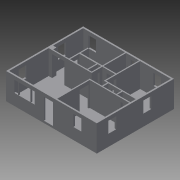
# Autodesk Inventor part: First Floor
Saved by Autodesk Inventor 2013 (Build 170138000, 138)
## iProperties
Created: 2013-06-17
Part Number: First Floor
Material: Generic
Document SubType Name: Modeling
Designer: Joey
Density: 1 g/cm^3
Author: Joey
Autodesk Inventor part; units mm, degrees
ref_plane "YZ Plane" through (0, 0, 0) normal (1, 0, 0) x (0, 1, 0)
ref_plane "XZ Plane" through (0, 0, 0) normal (0, 1, 0) x (-1, 0, 0)
ref_plane "XY Plane" through (0, 0, 0) normal (0, 0, 1) x (1, 0, 0)
sketch "Sketch1" plane through (0, 0, 0) normal (0, 1, 0) x (-1, 0, 0)
  line L0 (6400.8, 0) -> (-6400.8, 0) projected
  line L1 (4572, 3886.2) -> (4572, -3886.2)
  line L2 (4572, -3886.2) -> (-4572, -3886.2)
  line L3 (-4572, -3886.2) -> (-4572, 3886.2)
  line L4 (-4419.6, 3733.8) -> (-431.8, 3733.8)
  line L5 (-4419.6, 457.2) -> (-4419.6, 3733.8)
  line L6 (-4419.6, 3733.8) -> (-431.8, 3733.8)
  line L7 (-4419.6, 457.2) -> (-4419.6, 3733.8)
  line L8 (-4267.2, 342.9) -> (-4267.2, 457.2)
  line L9 (-3556, 457.2) -> (-3556, 342.9)
  line L10 (-4267.2, 342.9) -> (-4419.6, 342.9)
  line L11 (-431.8, 457.2) -> (-3556, 457.2)
  line L12 (-4267.2, 457.2) -> (-4419.6, 457.2)
  line L13 (-4419.6, -3733.8) -> (-1320.8, -3733.8)
  line L14 (-4419.6, -304.8) -> (-4419.6, -3733.8)
  line L15 (-4419.6, -3733.8) -> (-1320.8, -3733.8)
  line L16 (-4419.6, -304.8) -> (-4419.6, -3733.8)
  line L17 (-3098.8, 342.9) -> (-3098.8, -190.5)
  line L18 (-2679.7, -190.5) -> (-2679.7, -304.8)
  line L19 (-1968.5, -190.5) -> (-1968.5, -304.8)
  line L20 (-1663.7, -190.5) -> (-1663.7, 342.9)
  line L21 (-1549.4, -190.5) -> (-1549.4, 342.9)
  line L22 (-1320.8, -304.8) -> (-1968.5, -304.8)
  line L23 (-2679.7, -304.8) -> (-4419.6, -304.8)
  line L24 (-2984.5, -190.5) -> (-2984.5, 342.9)
  line L25 (-317.5, 342.9) -> (-1549.4, 342.9)
  line L26 (-1206.5, -190.5) -> (-1549.4, -190.5)
  line L27 (-1663.7, -190.5) -> (-1968.5, -190.5)
  line L28 (-1663.7, 342.9) -> (-2984.5, 342.9)
  line L29 (-3098.8, 342.9) -> (-3556, 342.9)
  line L30 (-2679.7, -190.5) -> (-2984.5, -190.5)
  line L31 (-3098.8, -190.5) -> (-4419.6, -190.5)
  line L32 (-1206.5, -3733.8) -> (88.9, -3733.8)
  line L33 (88.9, -3733.8) -> (88.9, -1447.8)
  line L34 (-1206.5, -1447.8) -> (-1206.5, -3733.8)
  line L35 (-1206.5, -3733.8) -> (88.9, -3733.8)
  line L36 (-1206.5, -1447.8) -> (-1206.5, -3733.8)
  line L37 (-1054.1, -1447.8) -> (-1054.1, -1333.5)
  line L38 (-342.9, -1447.8) -> (-342.9, -1333.5)
  line L39 (88.9, -1447.8) -> (-342.9, -1447.8)
  line L40 (-1054.1, -1447.8) -> (-1206.5, -1447.8)
  line L41 (88.9, -1333.5) -> (-342.9, -1333.5)
  line L42 (-1054.1, -1333.5) -> (-1206.5, -1333.5)
  line L43 (88.9, -1333.5) -> (88.9, -1079.5)
  line L44 (88.9, -1079.5) -> (203.2, -1079.5)
  line L45 (88.9, -254) -> (2857.5, -254)
  line L46 (762, 3733.8) -> (762, 3886.2)
  line L47 (-152.4, 3733.8) -> (-152.4, 3886.2)
  line L48 (546.1, -1333.5) -> (546.1, -368.3)
  line L49 (660.4, -1333.5) -> (660.4, -368.3)
  line L50 (2374.9, -1447.8) -> (203.2, -1447.8)
  line L51 (203.2, -3733.8) -> (203.2, -1447.8)
  line L52 (203.2, -1333.5) -> (203.2, -1079.5)
  line L53 (203.2, -1333.5) -> (546.1, -1333.5)
  line L54 (660.4, -1333.5) -> (2374.9, -1333.5)
  line L55 (546.1, -368.3) -> (203.2, -368.3)
  line L56 (203.2, -368.3) -> (203.2, -622.3)
  line L57 (203.2, -622.3) -> (88.9, -622.3)
  line L58 (88.9, -622.3) -> (88.9, -254)
  line L59 (2489.2, -2260.6) -> (2374.9, -2260.6)
  line L60 (2374.9, -2260.6) -> (2374.9, -1447.8)
  line L61 (4076.7, -254) -> (4076.7, -698.5)
  line L62 (4076.7, -698.5) -> (4419.6, -698.5)
  line L63 (4419.6, -698.5) -> (4419.6, -3733.8)
  line L64 (4419.6, 3733.8) -> (4419.6, -254)
  line L65 (-431.8, 1473.2) -> (-317.5, 1473.2)
  line L66 (-317.5, 558.8) -> (-431.8, 558.8)
  line L67 (-431.8, 3733.8) -> (-431.8, 1473.2)
  line L68 (-431.8, 558.8) -> (-431.8, 457.2)
  line L69 (-317.5, 3733.8) -> (-317.5, 1473.2)
  line L70 (-317.5, 558.8) -> (-317.5, 342.9)
  line L71 (-4419.6, 3733.8) -> (-431.8, 3733.8)
  line L72 (-317.5, 3733.8) -> (-152.4, 3733.8)
  line L73 (762, 3733.8) -> (4419.6, 3733.8)
  line L74 (-4572, 3886.2) -> (-152.4, 3886.2)
  line L75 (762, 3886.2) -> (4572, 3886.2)
  line L76 (4419.6, -3733.8) -> (203.2, -3733.8)
  line L77 (88.9, -3733.8) -> (-1206.5, -3733.8)
  line L78 (-1320.8, -3733.8) -> (-4419.6, -3733.8)
  line L79 (-4419.6, -3733.8) -> (-4419.6, -304.8)
  line L80 (-4419.6, -190.5) -> (-4419.6, 342.9)
  line L81 (-4419.6, 457.2) -> (-4419.6, 3733.8)
  line L82 (-1206.5, -3733.8) -> (-1206.5, -1447.8)
  line L83 (-1206.5, -419.1) -> (-1206.5, -190.5)
  line L84 (-1206.5, -1333.5) -> (-1320.8, -1333.5)
  line L85 (-1206.5, -419.1) -> (-1320.8, -419.1)
  line L86 (-1320.8, -3733.8) -> (-1320.8, -1333.5)
  line L87 (-1320.8, -419.1) -> (-1320.8, -304.8)
  line L88 (-342.9, -1333.5) -> (88.9, -1333.5)
  line L89 (88.9, -1447.8) -> (-342.9, -1447.8)
  line L90 (-342.9, -1447.8) -> (-342.9, -1333.5)
  line L91 (88.9, -1447.8) -> (88.9, -3733.8)
  line L92 (203.2, -3784.6) -> (203.2, -1447.8)
  line L93 (-1320.8, -3733.8) -> (-1320.8, -1333.5)
  line L94 (-1320.8, -1333.5) -> (-1206.5, -1333.5)
  line L95 (-1206.5, -1447.8) -> (-1206.5, -3733.8)
  line L96 (-1320.8, -1333.5) -> (-1054.1, -1333.5)
  line L97 (-1054.1, -1333.5) -> (-1054.1, -1447.8)
  line L98 (-1054.1, -1447.8) -> (-1206.5, -1447.8)
  line L99 (-1320.8, -1397) -> (-1320.8, -1333.5)
  line L100 (-4419.6, -3733.8) -> (-4572, -3733.8)
  line L101 (-4572, -3733.8) -> (-4572, -190.5)
  line L102 (-4419.6, -304.8) -> (-4419.6, -3733.8)
  line L103 (-2679.7, -190.5) -> (-2679.7, -304.8)
  line L104 (-2679.7, -304.8) -> (-4419.6, -304.8)
  line L105 (-4419.6, -304.8) -> (-4419.6, -190.5)
  line L106 (-4419.6, -190.5) -> (-3098.8, -190.5)
  line L107 (-2984.5, -190.5) -> (-2679.7, -190.5)
  line L108 (-431.8, 3733.8) -> (-4419.6, 3733.8)
  line L109 (2857.5, -368.3) -> (2857.5, -254)
  line L110 (4419.6, -254) -> (4076.7, -254)
  line L111 (2489.2, -2260.6) -> (2489.2, -1333.5)
  line L112 (2374.9, -1333.5) -> (2374.9, -368.3)
  line L113 (2489.2, -368.3) -> (2489.2, -1333.5)
  line L114 (2857.5, -368.3) -> (2489.2, -368.3)
  line L115 (2374.9, -368.3) -> (660.4, -368.3)
  point P0 (0, 0)
  point P1 (-1663.7, -304.8)
  dimension "d0" = 7772.4
  dimension "d2" = 9144
  dimension "d3" = 7467.6
  dimension "d11" = 711.2
  dimension "d19" = 711.2
  dimension "d21" = 114.3
  dimension "d22" = 114.3
  dimension "d29" = 711.2
  dimension "d34" = 3810
  dimension "d35" = 914.4
  dimension "d40" = 114.3
  dimension "d42" = 114.3
  dimension "d48" = 114.3
  dimension "d52" = 114.3
  dimension "d61" = 114.3
  dimension "d117" = 152.4
  dimension "d118" = 152.4
  dimension "d119" = 152.4
  dimension "d120" = 152.4
  dimension "d121" = 152.4
  dimension "d122" = 152.4
  dimension "d123" = 152.4
  dimension "d124" = 114.3
  dimension "d125" = 114.3
  dimension "d126" = 114.3
  dimension "d127" = 114.3
  dimension "d128" = 114.3
  dimension "d129" = 114.3
  dimension "d131" = 114.3
  dimension "d133" = 114.3
  dimension "d134" = 114.3
  dimension "d135" = 152.4
  dimension "d138" = 152.4
  dimension "d139" = 3429
  dimension "d140" = 3276.6
  dimension "d141" = 3276.6
  dimension "d142" = 3987.8
  dimension "d148" = 4216.4
  dimension "d149" = 114.3
  dimension "d154" = 457.2
  dimension "d155" = 254
  dimension "d160" = 342.9
  dimension "d162" = 1320.8
  dimension "d164" = 304.8
  dimension "d165" = 1320.8
  dimension "d166" = 152.4
  dimension "d170" = 114.3
  dimension "d172" = 914.4
  dimension "d173" = 152.4
  dimension "d174" = 914.4
  dimension "d175" = 114.3
  dimension "d176" = 114.3
  dimension "d177" = 3098.8
  dimension "d238" = 3911.6
  dimension "d241" = 3479.8
  dimension "d243" = 1219.2
  dimension "d246" = 444.5
  dimension "d247" = 1714.5
  dimension "d248" = 965.2
  constraints: 230 end point, 62 parallel, 58 perpendicular, 16 horizontal, 13 collinear, 3 point on line
  measures "d0" distance of L2.end L3.end
  measures "d2" distance of L1.end L2.end
  measures "d3" distance of L13.start L4.start
  measures "d11" distance between parallel lines of L8 L9
  measures "d19" distance between parallel lines of L18 L19
  measures "d21" distance between parallel lines of L20 L21
  measures "d22" distance between parallel lines of L17 L24
  measures "d29" distance between parallel lines of L37 L38
  measures "d34" distance between parallel lines of L1 L46
  measures "d35" distance between parallel lines of L46 L47
  measures "d40" distance between parallel lines of L41 L39
  measures "d42" distance of L45.end L109.start
  measures "d48" distance between parallel lines of L45 L55
  measures "d52" distance of L59.start L59.end
  measures "d61" distance between parallel lines of L69 L67
  measures "d117" distance between parallel lines of L74 L4
  measures "d118" distance between parallel lines of L2 L76
  measures "d119" distance between parallel lines of L75 L73
  measures "d120" distance between parallel lines of L2 L32
  measures "d121" distance between parallel lines of L3 L14
  measures "d122" distance between parallel lines of L64 L1
  measures "d123" distance between parallel lines of L3 L5
  measures "d124" distance between parallel lines of L25 L11
  measures "d125" distance between parallel lines of L11 L28
  measures "d126" distance between parallel lines of L31 L23
  measures "d127" distance between parallel lines of L12 L10
  measures "d128" distance between parallel lines of L26 L22
  measures "d129" distance between parallel lines of L22 L27
  measures "d131" distance from line of L43.end L52
  measures "d133" distance between parallel lines of L54 L50
  measures "d134" distance between parallel lines of L48 L49
  measures "d135" distance between parallel lines of L1 L63
  measures "d138" distance between parallel lines of L74 L72
  measures "d139" distance between parallel lines of L13 L23
  measures "d140" distance between parallel lines of L4 L11
  measures "d141" distance between parallel lines of L4 L12
  measures "d142" distance between parallel lines of L5 L67
  measures "d148" distance between parallel lines of L63 L51
  measures "d149" distance between parallel lines of L51 L33
  measures "d154" distance between parallel lines of L57 L44
  measures "d155" distance between parallel lines of L55 L57
  measures "d160" distance between parallel lines of L83 L21
  measures "d162" distance between parallel lines of L80 L17
  measures "d164" distance between parallel lines of L20 L19
  measures "d165" distance between parallel lines of L20 L24
  measures "d166" distance between parallel lines of L5 L8
  measures "d170" distance between parallel lines of L70 L68
  measures "d172" distance between parallel lines of L84 L85
  measures "d173" distance between parallel lines of L37 L83
  measures "d174" distance between parallel lines of L66 L65
  measures "d175" distance between parallel lines of L83 L87
  measures "d176" distance between parallel lines of L34 L86
  measures "d177" distance between parallel lines of L86 L14
  measures "d238" distance between parallel lines of L1 L49
  measures "d241" distance between parallel lines of L76 L45
  measures "d243" distance between parallel lines of L109 L61
  measures "d246" distance between parallel lines of L62 L110
  measures "d247" distance between parallel lines of L49 L112
  measures "d248" distance between parallel lines of L54 L115
extrude "Extrusion8" add sketch "Sketch1" along normal blind 2438.4 contours L1 L2 L3 L100 L13 L86 L84 L42 L37 L40 L34 L32 L33 L39 L38 L41 L43 L44 L52 L53 L48 L55 L56 L57 L58 L45 L109 L114 L113 L111 L59 L60 L50 L51 L76 L63 L62 L61 L110 L64 L0 | L0 L64 L73 L46 L75 L1 | L21 L26 L83 L85 L87 L22 L19 L27 L20 L0 | L0 L20 L28 L24 L17 L29 L9 L11 L68 L66 L70 L25 L21 | L3 L0 L80 L105 L14 L100 | L24 L30 L18 L23 L105 L31 L17 L0 | L3 L74 L47 L72 L69 L65 L67 L4 L5 L12 L8 L10 L80 L0 | L49 L115 L112 L54
sketch "Sketch10" plane through (4572, 2438.4, 3886.2) normal (1, 0, 0) x (0, 0, -1)
  line L0 (7772.4, -2438.4) -> (7772.4, 0) projected
  line L1 (0, 0) -> (7772.4, 0) projected
  line L2 (0, -2438.4) -> (0, 0) projected
  line L3 (4699, -355.6) -> (5486.4, -355.6)
  line L4 (5486.4, -355.6) -> (5486.4, -1498.6)
  line L5 (5486.4, -1498.6) -> (4699, -1498.6)
  line L6 (4699, -1498.6) -> (4699, -355.6)
  line L7 (1168.4, -355.6) -> (1955.8, -355.6)
  line L8 (1955.8, -355.6) -> (1955.8, -1498.6)
  line L9 (1955.8, -1498.6) -> (1168.4, -1498.6)
  line L10 (1168.4, -1498.6) -> (1168.4, -355.6)
  point P0 (7772.4, -2641.6)
  point P1 (0, -2641.6)
  point P2 (3886.2, -2438.4)
  dimension "d184" = 355.6
  dimension "d185" = 1168.4
  dimension "d186" = 787.4
  dimension "d187" = 1143
  dimension "d188" = 1143
  dimension "d189" = 787.4
  dimension "d190" = 2286
  constraints: 16 end point, 4 parallel, 2 horizontal, 2 perpendicular, 1 collinear
  measures "d184" distance between parallel lines of L1 L7
  measures "d185" distance between parallel lines of L2 L10
  measures "d186" distance between parallel lines of L10 L8
  measures "d187" distance between parallel lines of L9 L7
  measures "d188" distance between parallel lines of L3 L5
  measures "d189" distance between parallel lines of L4 L6
  measures "d190" distance between parallel lines of L0 L4
extrude "Extrusion11" cut sketch "Sketch10" against normal blind 152.4
sketch "Sketch11" plane through (-4572, 2438.4, 3886.2) normal (0, 0, 1) x (1, 0, 0)
  line L0 (9144, -2438.4) -> (9144, 0) projected
  line L1 (0, -2438.4) -> (0, 0) projected
  line L2 (6781.8, -355.6) -> (7569.2, -355.6)
  line L3 (7569.2, -355.6) -> (7569.2, -1498.6)
  line L4 (7569.2, -1498.6) -> (6781.8, -1498.6)
  line L5 (6781.8, -1498.6) -> (6781.8, -355.6)
  line L6 (774.7, -355.6) -> (2933.7, -355.6)
  line L7 (2933.7, -355.6) -> (2933.7, -1498.6)
  line L8 (2933.7, -1498.6) -> (774.7, -1498.6)
  line L9 (774.7, -1498.6) -> (774.7, -355.6)
  line L10 (1257.3, -355.6) -> (2451.1, -355.6)
  line L11 (2451.1, -355.6) -> (2451.1, -1498.6)
  line L12 (2451.1, -1498.6) -> (1257.3, -1498.6)
  line L13 (1257.3, -1498.6) -> (1257.3, -355.6)
  line L14 (825.5, -355.6) -> (1206.5, -355.6)
  line L15 (1206.5, -355.6) -> (1206.5, -1498.6)
  line L16 (1206.5, -1498.6) -> (825.5, -1498.6)
  line L17 (825.5, -1498.6) -> (825.5, -355.6)
  line L18 (1257.3, -355.6) -> (2451.1, -355.6)
  line L19 (2451.1, -355.6) -> (2451.1, -1498.6)
  line L20 (2451.1, -1498.6) -> (1257.3, -1498.6)
  line L21 (1257.3, -1498.6) -> (1257.3, -355.6)
  line L22 (2501.9, -355.6) -> (2882.9, -355.6)
  line L23 (2882.9, -355.6) -> (2882.9, -1498.6)
  line L24 (2882.9, -1498.6) -> (2501.9, -1498.6)
  line L25 (2501.9, -1498.6) -> (2501.9, -355.6)
  line L26 (4724.4, 0) -> (9144, 0) projected
  point P0 (9144, -2641.6)
  point P1 (0, -2641.6)
  point P2 (4572, -2438.4)
  dimension "d193" = 1574.8
  dimension "d194" = 787.4
  dimension "d195" = 1143
  dimension "d196" = 1193.8
  dimension "d197" = 2159
  dimension "d199" = 482.6
  dimension "d200" = 774.7
  dimension "d203" = 50.8
  dimension "d204" = 50.8
  dimension "d205" = 0
  dimension "d206" = 0
  dimension "d207" = 0
  dimension "d208" = 0
  dimension "d209" = 50.8
  dimension "d210" = 50.8
  dimension "d252" = 355.6
  constraints: 48 end point, 12 parallel, 8 collinear, 6 horizontal, 6 perpendicular
  measures "d193" distance between parallel lines of L0 L3
  measures "d194" distance between parallel lines of L3 L5
  measures "d195" distance between parallel lines of L2 L4
  measures "d196" distance of L11.end L12.end
  measures "d197" distance between parallel lines of L7 L9
  measures "d199" distance between parallel lines of L9 L13
  measures "d200" distance between parallel lines of L1 L9
  measures "d203" distance between parallel lines of L13 L15
  measures "d204" distance between parallel lines of L9 L17
  measures "d205" distance between parallel lines of L6 L14
  measures "d206" distance between parallel lines of L8 L16
  measures "d207" distance between parallel lines of L11 L19
  measures "d208" distance between parallel lines of L13 L21
  measures "d209" distance between parallel lines of L7 L23
  measures "d210" distance between parallel lines of L11 L25
  measures "d252" distance between parallel lines of L26 L2
extrude "Extrusion12" cut sketch "Sketch11" against normal blind 152.4 contours L2 L3 L4 L5 | L6 L15 L8 L17 | L6 L11 L8 L13 | L6 L23 L8 L25
sketch "Sketch12" plane through (-4572, 2438.4, -3886.2) normal (-1, 0, 0) x (0, 0, 1)
  line L0 (7772.4, -2438.4) -> (7772.4, 0) projected
  line L1 (0, 0) -> (7772.4, 0) projected
  line L2 (0, -2438.4) -> (0, 0) projected
  line L3 (1905, -355.6) -> (2692.4, -355.6)
  line L4 (2692.4, -355.6) -> (2692.4, -1498.6)
  line L5 (2692.4, -1498.6) -> (1905, -1498.6)
  line L6 (1905, -1498.6) -> (1905, -355.6)
  line L7 (5880.1, -355.6) -> (6667.5, -355.6)
  line L8 (6667.5, -355.6) -> (6667.5, -1498.6)
  line L9 (6667.5, -1498.6) -> (5880.1, -1498.6)
  line L10 (5880.1, -1498.6) -> (5880.1, -355.6)
  point P0 (7772.4, -2641.6)
  point P1 (0, -2641.6)
  point P2 (3886.2, -2438.4)
  dimension "d213" = 355.6
  dimension "d214" = 787.4
  dimension "d215" = 787.4
  dimension "d216" = 1143
  dimension "d217" = 1104.9
  dimension "d218" = 1905
  constraints: 16 end point, 4 parallel, 2 collinear, 2 horizontal, 2 perpendicular
  measures "d213" distance between parallel lines of L1 L7
  measures "d214" distance between parallel lines of L6 L4
  measures "d215" distance between parallel lines of L8 L10
  measures "d216" distance between parallel lines of L5 L3
  measures "d217" distance between parallel lines of L0 L8
  measures "d218" distance between parallel lines of L2 L6
extrude "Extrusion13" cut sketch "Sketch12" against normal blind 152.4
sketch "Sketch13" plane through (4572, 2438.4, -3886.2) normal (0, 0, -1) x (-1, 0, 0)
  line L0 (9144, -2438.4) -> (9144, 0) projected
  line L1 (0, 0) -> (9144, 0) projected
  line L2 (0, -2438.4) -> (0, 0) projected
  line L3 (1143, -355.6) -> (1905, -355.6)
  line L4 (1905, -355.6) -> (1905, -1498.6)
  line L5 (1905, -1498.6) -> (1143, -1498.6)
  line L6 (1143, -1498.6) -> (1143, -355.6)
  line L7 (7696.2, -355.6) -> (8458.2, -355.6)
  line L8 (8458.2, -355.6) -> (8458.2, -1498.6)
  line L9 (8458.2, -1498.6) -> (7696.2, -1498.6)
  line L10 (7696.2, -1498.6) -> (7696.2, -355.6)
  line L11 (3810, -355.6) -> (4216.4, -355.6)
  line L12 (4216.4, -355.6) -> (4216.4, -1016)
  line L13 (4216.4, -1016) -> (3810, -1016)
  line L14 (3810, -1016) -> (3810, -355.6)
  point P0 (9144, -2641.6)
  point P1 (0, -2641.6)
  point P2 (4572, -2438.4)
  dimension "d221" = 762
  dimension "d223" = 355.6
  dimension "d224" = 1143
  dimension "d225" = 685.8
  dimension "d226" = 762
  dimension "d227" = 1143
  dimension "d228" = 406.4
  dimension "d229" = 660.4
  dimension "d230" = 3810
  constraints: 24 end point, 6 parallel, 3 collinear, 3 horizontal, 3 perpendicular
  measures "d221" distance between parallel lines of L6 L4
  measures "d223" distance between parallel lines of L1 L3
  measures "d224" distance between parallel lines of L2 L6
  measures "d225" distance between parallel lines of L0 L8
  measures "d226" distance between parallel lines of L8 L10
  measures "d227" distance between parallel lines of L9 L7
  measures "d228" distance between parallel lines of L14 L12
  measures "d229" distance between parallel lines of L11 L13
  measures "d230" distance between parallel lines of L2 L14
extrude "Extrusion14" cut sketch "Sketch13" against normal blind 152.4
sketch "Sketch14" plane through (0, 0, 0) normal (0, -1, 0) x (1, 0, 0)
  line L0 (-546.1, -368.3) -> (-546.1, -1333.5) projected
  line L1 (-2489.2, -2260.6) -> (-2489.2, -368.3) projected
  line L2 (-660.4, -368.3) -> (-2489.2, -368.3)
  line L3 (-2489.2, -368.3) -> (-2489.2, -1314.45)
  line L4 (-2489.2, -1314.45) -> (-660.4, -1314.45)
  line L5 (-660.4, -1314.45) -> (-660.4, -368.3)
  point P0 (0, 0)
  dimension "d249" = 114.3
  constraints: 8 end point, 2 parallel, 1 collinear, 1 horizontal, 1 perpendicular
  measures "d249" distance between parallel lines of L0 L5
extrude "Extrusion15" cut sketch "Sketch14" against normal blind 2438.4
sketch "Sketch15" plane through (0, 2438.4, 0) normal (0, 1, 0) x (1, 0, 0)
  line L0 (-4076.7, 254) -> (-2857.5, 254)
  line L1 (-2857.5, 254) -> (-2857.5, 368.3)
  line L2 (-2857.5, 368.3) -> (-4076.7, 368.3)
  line L3 (-4076.7, 368.3) -> (-4076.7, 254)
  line L4 (-203.2, 622.3) -> (-88.9, 622.3)
  line L5 (-88.9, 622.3) -> (-88.9, 1079.5)
  line L6 (-88.9, 1079.5) -> (-203.2, 1079.5)
  line L7 (-203.2, 1079.5) -> (-203.2, 622.3)
  line L8 (317.5, -558.8) -> (431.8, -558.8)
  line L9 (431.8, -558.8) -> (431.8, -1473.2)
  line L10 (431.8, -1473.2) -> (317.5, -1473.2)
  line L11 (317.5, -1473.2) -> (317.5, -558.8)
  line L12 (1968.5, 190.5) -> (2679.7, 190.5)
  line L13 (2679.7, 190.5) -> (2679.7, 304.8)
  line L14 (2679.7, 304.8) -> (1968.5, 304.8)
  line L15 (1968.5, 304.8) -> (1968.5, 190.5)
  line L16 (1206.5, 419.1) -> (1320.8, 419.1)
  line L17 (1320.8, 419.1) -> (1320.8, 1333.5)
  line L18 (1320.8, 1333.5) -> (1206.5, 1333.5)
  line L19 (1206.5, 1333.5) -> (1206.5, 419.1)
  line L20 (1054.1, 1333.5) -> (342.9, 1333.5)
  line L21 (342.9, 1333.5) -> (342.9, 1447.8)
  line L22 (342.9, 1447.8) -> (1054.1, 1447.8)
  line L23 (1054.1, 1447.8) -> (1054.1, 1333.5)
  line L24 (3556, -342.9) -> (4267.2, -342.9)
  line L25 (4267.2, -342.9) -> (4267.2, -457.2)
  line L26 (4267.2, -457.2) -> (3556, -457.2)
  line L27 (3556, -457.2) -> (3556, -342.9)
  line L28 (152.4, -3886.2) -> (-762, -3886.2)
  line L29 (-762, -3886.2) -> (-762, -3733.8)
  line L30 (-762, -3733.8) -> (152.4, -3733.8)
  line L31 (152.4, -3733.8) -> (152.4, -3886.2)
  point P0 (0, 0)
  constraints: 64 end point, 16 parallel, 8 horizontal, 8 perpendicular
extrude "Extrusion16" add sketch "Sketch15" against normal blind 355.6 contours L3 L2 L1 L0 | L8 L9 L10 L11 | L15 L14 L13 L12 | L19 L18 L17 L16 | L20 L21 L22 L23 | L24 L25 L26 L27 | L28 L29 L30 L31
sketch "Sketch16" plane through (0, 0, 0) normal (0, -1, 0) x (1, 0, 0)
  line L0 (-660.4, -1314.45) -> (-2489.2, -1314.45) projected
  line L1 (-4572, 3886.2) -> (4572, 3886.2)
  line L2 (4572, 3886.2) -> (4572, -3886.2)
  line L3 (4572, -3886.2) -> (-4572, -3886.2)
  line L4 (-4572, -3886.2) -> (-4572, 3886.2)
  line L5 (-660.4, -368.3) -> (-2374.9, -368.3)
  line L6 (-2374.9, -368.3) -> (-2374.9, -1314.45)
  line L7 (-2374.9, -1314.45) -> (-660.4, -1314.45)
  line L8 (-660.4, -1314.45) -> (-660.4, -368.3)
  point P0 (0, 0)
  constraints: 16 end point, 4 parallel, 2 horizontal, 2 perpendicular, 1 point on line
extrude "Extrusion17" add sketch "Sketch16" along normal blind 203.2
sketch "Sketch17" plane through (0, 2438.4, 0) normal (0, 1, 0) x (1, 0, 0)
  line L0 (-203.2, 1079.5) -> (-88.9, 1079.5)
  line L1 (-88.9, 1079.5) -> (-88.9, 622.3)
  line L2 (-88.9, 622.3) -> (-203.2, 622.3)
  line L3 (-203.2, 622.3) -> (-203.2, 1079.5)
  point P0 (0, 0)
  constraints: 8 end point, 2 parallel, 1 horizontal, 1 perpendicular
extrude "Extrusion18" add sketch "Sketch17" against normal blind 355.6
sketch "Sketch18" plane through (0, 2438.4, 0) normal (0, 1, 0) x (1, 0, 0)
  line L0 (-660.4, 368.3) -> (-4076.7, 368.3) projected
  line L1 (-2489.2, 1314.45) -> (-660.4, 1314.45) projected
  line L2 (-2374.9, 368.3) -> (-2374.9, 1314.45) projected
  line L3 (-2489.2, 1314.45) -> (-2374.9, 1314.45)
  line L4 (-2374.9, 1314.45) -> (-2374.9, 1200.15)
  line L5 (-2374.9, 1200.15) -> (-2489.2, 1200.15)
  line L6 (-2489.2, 1200.15) -> (-2489.2, 1314.45)
  line L7 (-2489.2, 368.3) -> (-2374.9, 368.3)
  line L8 (-2374.9, 368.3) -> (-2374.9, 482.6)
  line L9 (-2374.9, 482.6) -> (-2489.2, 482.6)
  line L10 (-2489.2, 482.6) -> (-2489.2, 368.3)
  line L11 (-2489.2, 482.6) -> (-2374.9, 482.6)
  line L12 (-2374.9, 482.6) -> (-2374.9, 1200.15)
  line L13 (-2374.9, 1200.15) -> (-2489.2, 1200.15)
  line L14 (-2489.2, 1200.15) -> (-2489.2, 482.6)
  line L15 (-2489.2, 482.6) -> (-2374.9, 482.6)
  line L16 (-2374.9, 482.6) -> (-2374.9, 368.3)
  line L17 (-2374.9, 368.3) -> (-2489.2, 368.3)
  line L18 (-2489.2, 368.3) -> (-2489.2, 482.6)
  line L19 (-2489.2, 368.3) -> (-2374.9, 368.3)
  line L20 (-2374.9, 368.3) -> (-2374.9, 1314.45)
  line L21 (-2374.9, 1314.45) -> (-2489.2, 1314.45)
  line L22 (-2489.2, 1314.45) -> (-2489.2, 368.3)
  point P0 (0, 0)
  dimension "d259" = 114.3
  dimension "d260" = 114.3
  constraints: 40 end point, 10 parallel, 5 horizontal, 5 perpendicular, 3 point on line
  measures "d259" distance between parallel lines of L1 L5
  measures "d260" distance between parallel lines of L0 L9
extrude "Extrusion19" add sketch "Sketch18" against normal blind 355.6 contours L9 L14 L5 L2
extrude "Extrusion20" add sketch "Sketch18" against normal blind 2438.4 contours L0 L10 L9 L2 | L5 L6 L1 L2
body "Solid2"
